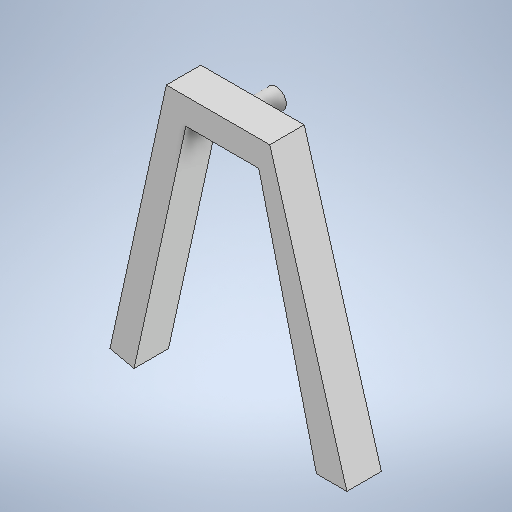
# Autodesk Inventor part: F stand
Saved by Autodesk Inventor 2025.1 (Build 291241000, 241)
## iProperties
Created: 2025-04-20
Part Number: F stand
Material: Generic
Document SubType Name: Modeling
Designer: POORNIMA HIREMATH
Density: 1 g/cm^3
Appearance: Default
Author: POORNIMA HIREMATH
Autodesk Inventor part; units mm, degrees
ref_plane "YZ Plane" through (0, 0, 0) normal (1, 0, 0) x (0, 1, 0)
ref_plane "XZ Plane" through (0, 0, 0) normal (0, 1, 0) x (-1, 0, 0)
ref_plane "XY Plane" through (0, 0, 0) normal (0, 0, 1) x (1, 0, 0)
sketch "Sketch1" plane through (0, 0, 0) normal (0, 0, 1) x (1, 0, 0)
  line L0 (-5.1167, 18.7008) -> (-12.6322, -15.4828)
  line L1 (-12.6322, -15.4828) -> (-16.1242, -14.715)
  line L2 (-16.1242, -14.715) -> (-7.9505, 22.4623)
  line L3 (-7.9505, 22.4623) -> (7.0495, 22.4623)
  line L4 (7.0495, 22.4623) -> (18.2297, -15.4828)
  line L5 (18.2297, -15.4828) -> (13.8247, -15.4828)
  line L6 (13.8247, -15.4828) -> (5.4553, 18.7008)
  line L7 (5.4553, 18.7008) -> (-5.1167, 18.7008)
  point P0 (0, 0)
  dimension "d0" = 35
  dimension "d1" = 15
  constraints: 16 end point, 2 parallel, 2 perpendicular, 1 horizontal
  measures "d0" distance of L0.start L0.end
  measures "d1" distance of L2.end L3.end
extrude "Extrusion1" add sketch "Sketch1" along normal blind 5
sketch "Sketch2" plane through (0, 0, 0) normal (0, 0, -1) x (-1, 0, 0)
  circle A0 centre (0, 20.7839) radius 1.45
  point P0 (0, 0)
  dimension "d4" = 2.9
  constraints: 1 centre point
  measures "d4" diameter of A0
extrude "Extrusion2" add sketch "Sketch2" along normal blind 3
body "Solid1"
